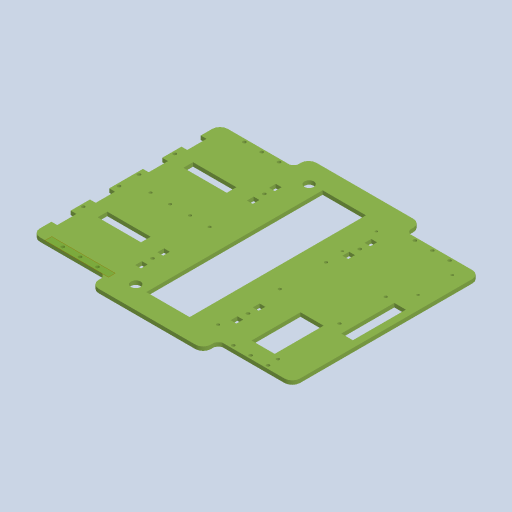
# Autodesk Inventor part: верхняя пластина
Saved by Autodesk Inventor 2024.2 (Build 282272000, 272)
## iProperties
Created: 2025-11-23
Part Number: верхняя пластина
Material: Типовые
Document SubType Name: Modeling
Designer: katya_notebook
Density: 1 g/cm^3
Appearance: Оливково-зеленый
Mass: 177.745 g
Surface Area: 959.322 cm^2
Volume: 177.745 cm^3
Author: katya_notebook
Autodesk Inventor part; units mm, degrees
ref_plane "YZ Plane" through (0, 0, 0) normal (1, 0, 0) x (0, 1, 0)
ref_plane "XZ Plane" through (0, 0, 0) normal (0, 1, 0) x (-1, 0, 0)
ref_plane "XY Plane" through (0, 0, 0) normal (0, 0, 1) x (1, 0, 0)
ref_plane "РабПлоскость1" through (-487.5503, -280.3956, -187.6025) normal (0, -1, 0) x (1, 0, 0)
sketch "Эскиз1" plane through (-487.5503, -280.3956, -187.6025) normal (0, -1, 0) x (1, 0, 0)
  line L0 (-76.4763, 6.5) -> (193.5237, 6.5)
  line L1 (193.5237, 6.5) -> (193.5237, -188.5)
  line L2 (193.5237, -188.5) -> (-76.4763, -188.5)
  line L3 (-76.4763, -188.5) -> (-76.4763, 6.5)
  line L4 (-76.4763, -13.5) -> (-76.4763, -1.5) projected
  circle A0 centre (-12, 3.25) radius 1.75
  circle A1 centre (-48, 3.25) radius 1.75
  circle A2 centre (-30, 3.25) radius 1.75
  line L5 (-76.4763, -91) -> (193.5237, -91)
  circle A3 centre (-12, -185.25) radius 1.75
  circle A4 centre (-48, -185.25) radius 1.75
  circle A5 centre (-30, -185.25) radius 1.75
  point P0 (487.5503, 187.6025)
  point P1 (-60, 3.25)
  dimension "d0" = 195
  dimension "d1" = 270
  dimension "d2" = 0
  dimension "d5" = 3.5
  dimension "d6" = 3.5
  dimension "d8" = 12
  dimension "d9" = 3.25
  dimension "d10" = 3.25
  dimension "d11" = 3.5
  dimension "d12" = 3.25
  dimension "d13" = 18
  dimension "d14" = 97.5
  constraints: 10 end point, 6 centre point, 3 symmetric about line, 2 parallel, 2 perpendicular, 1 horizontal, 1 midpoint, 1 point on line, 3 other
  measures "d0" distance of L0.end L1.end
  measures "d1" distance of L1.end L2.end
  measures "d2" distance between parallel lines of L4 L3
  measures "d5" diameter of A1
  measures "d6" diameter of A0
  measures "d8" distance of A1.centre point (-60, 3.25)
  measures "d9" distance from line of L0 A0.centre
  measures "d10" distance from line of L0 A1.centre
  measures "d11" diameter of A2
  measures "d12" distance from line of L0 A2.centre
  measures "d13" distance of A1.centre A2.centre
  measures "d14" distance between parallel lines of L5 L0
extrude "Выдавливание1" add sketch "Эскиз1" along normal blind 4 contours L0 L1 L5 L3 | L1 L2 L3 L5 | A0 | A1 | A2 | A3 | A4 | A5
sketch "Эскиз2" plane through (-487.5503, -284.3956, -187.6025) normal (0, -1, 0) x (1, 0, 0)
  circle A0 centre (-48, -185.25) radius 1.75 projected
  circle A1 centre (-30, -185.25) radius 1.75 projected
  circle A2 centre (-12, -185.25) radius 1.75 projected
  line L0 (0, -182) -> (-60, -182) projected
  line L1 (-60, -182) -> (-60, -188.5) projected
  line L2 (0, -188.5) -> (-60, -188.5) projected
  line L3 (0, -182) -> (0, -188.5) projected
  circle A3 centre (-48, 3.25) radius 1.75 projected
  circle A4 centre (-30, 3.25) radius 1.75 projected
  circle A5 centre (-12, 3.25) radius 1.75 projected
  line L4 (0, 0) -> (-60, 0) projected
  line L5 (0, 0) -> (0, 6.5) projected
  line L6 (0, 6.5) -> (-60, 6.5) projected
  line L7 (-60, 0) -> (-60, 6.5) projected
  circle A6 centre (165.0475, 3.25) radius 1.75 projected
  circle A7 centre (129.0475, 3.25) radius 1.75 projected
  circle A8 centre (147.0475, 3.25) radius 1.75 projected
  line L8 (116.803, 6.5) -> (116.803, 0) projected
  line L9 (116.803, 0) -> (176.803, 0) projected
  line L10 (176.803, 0) -> (176.803, 6.5) projected
  line L11 (176.803, 6.5) -> (116.803, 6.5) projected
  circle A9 centre (165.0475, -185.25) radius 1.75 projected
  circle A10 centre (129.0475, -185.25) radius 1.75 projected
  circle A11 centre (147.0475, -185.25) radius 1.75 projected
  line L12 (116.803, -188.5) -> (116.803, -182) projected
  line L13 (176.803, -188.5) -> (116.803, -188.5) projected
  line L14 (176.803, -182) -> (176.803, -188.5) projected
  line L15 (116.803, -182) -> (176.803, -182) projected
  line L16 (81.0237, 0.5) -> (81.0237, -182.5) projected
  line L17 (36.0237, 0.5) -> (81.0237, 0.5) projected
  line L18 (36.0237, -182.5) -> (36.0237, 0.5) projected
  line L19 (36.0237, -182.5) -> (81.0237, -182.5) projected
  point P0 (487.5503, 187.6025)
extrude "Выдавливание2" cut sketch "Эскиз2" against normal blind 10 contours A0 | A1 | A2 | A3 | A4 | A5 | A6 | A7 | A8 | A9 | A10 | A11
sketch "Эскиз3" plane through (-487.5503, -284.3956, -187.6025) normal (0, -1, 0) x (1, 0, 0)
  circle A0 centre (23.5237, -1) radius 5 projected
  circle A1 centre (23.5237, -181) radius 5 projected
  line L0 (36.0237, -182.5) -> (36.0237, 0.5) projected
  line L1 (81.0237, 0.5) -> (81.0237, -182.5) projected
  line L2 (36.0237, 0.5) -> (81.0237, 0.5) projected
  line L3 (81.0237, -182.5) -> (36.0237, -182.5) projected
  point P0 (487.5503, 187.6025)
extrude "Выдавливание3" cut sketch "Эскиз3" against normal blind 10
sketch "Эскиз4" plane through (-487.5503, -284.3956, -187.6025) normal (0, -1, 0) x (1, 0, 0)
  arc A0 (116.803, 10.7701) -> (120.803, 6.5) centre (124.2371, 13.7254) ccw projected
  line L0 (116.803, 10.7701) -> (0.2701, 10.7701) projected
  arc A1 (-4, 6.5) -> (0.2701, 10.7701) centre (-7.1034, 13.8735) ccw projected
  arc A2 (0, -192.5) -> (-4, -188.5) centre (-7.2915, -195.7915) ccw projected
  line L1 (0, -192.5) -> (116.803, -192.5) projected
  arc A3 (120.803, -188.5) -> (116.803, -192.5) centre (124.0945, -195.7915) ccw projected
  line L2 (120.803, -188.5) -> (-4, -188.5)
  line L3 (-4, 6.5) -> (120.803, 6.5)
  point P0 (487.5503, 187.6025)
  constraints: 4 end point, 1 horizontal, 1 parallel
extrude "Выдавливание4" add sketch "Эскиз4" against normal blind 4
sketch "Эскиз5" plane through (-487.5503, -284.3956, -187.6025) normal (0, -1, 0) x (1, 0, 0)
  line L0 (174.5237, -118.4235) -> (174.5237, -63.4235) projected
  line L1 (186.5237, -118.4235) -> (174.5237, -118.4235) projected
  line L2 (186.5237, -63.4235) -> (186.5237, -118.4235) projected
  line L3 (174.5237, -63.4235) -> (186.5237, -63.4235) projected
  point P0 (487.5503, 187.6025)
extrude "Выдавливание5" cut sketch "Эскиз5" against normal blind 10
ref_plane "РабПлоскость2" through (-558.0266, -285.3956, -376.1025) normal (1, 0, 0) x (0, 1, 0)
sketch "Эскиз7" plane through (-564.0266, -280.3956, -376.1025) normal (-1, 0, 0) x (0, 0, 1)
  line L0 (175, -5) -> (175, 0) projected
  line L1 (155, 0) -> (155, -5) projected
  line L2 (155, -5) -> (175, -5) projected
  line L3 (195, 0) -> (0, 0) projected
  line L4 (115, -5) -> (135, -5) projected
  line L5 (135, -5) -> (135, 0) projected
  line L6 (115, 0) -> (115, -5) projected
  line L7 (80, -5) -> (80, 0) projected
  line L8 (60, -5) -> (80, -5) projected
  line L9 (60, 0) -> (60, -5) projected
  line L10 (40, -5) -> (40, 0) projected
  line L11 (20, -5) -> (40, -5) projected
  line L12 (20, 0) -> (20, -5) projected
  line L13 (90.375, 55.705) -> (90.375, 55.205) projected
  line L14 (90.375, 55.205) -> (88.875, 55.205) projected
  line L15 (85.375, 55.205) -> (83.875, 55.205) projected
  line L16 (83.875, 55.205) -> (83.875, 55.705) projected
  line L17 (80, 59.705) -> (80, 60.705) projected
  line L18 (80, 60.705) -> (60, 60.705) projected
  line L19 (60, 60.705) -> (60, 59.705) projected
  line L20 (51.75, 55.205) -> (51.75, 47.705) projected
  line L21 (53.25, 55.705) -> (53.25, 55.205) projected
  line L22 (53.25, 55.205) -> (51.75, 55.205) projected
  line L23 (51.75, 47.705) -> (48.25, 47.705) projected
  line L24 (48.25, 47.705) -> (48.25, 55.205) projected
  line L25 (48.25, 55.205) -> (46.75, 55.205) projected
  line L26 (46.75, 55.205) -> (46.75, 55.705) projected
  line L27 (40, 59.705) -> (40, 60.705) projected
  line L28 (40, 60.705) -> (20, 60.705) projected
  line L29 (20, 60.705) -> (20, 59.705) projected
  line L30 (0, 59.705) -> (0, 0) projected
  line L31 (20, 0) -> (0, 0) projected
  line L32 (20, 0) -> (20, -5) projected
  line L33 (20, -5) -> (40, -5) projected
  line L34 (40, -5) -> (40, 0) projected
  line L35 (48.25, 0) -> (40, 0) projected
  line L36 (48.25, 0) -> (48.25, 1.5) projected
  line L37 (48.25, 1.5) -> (46.75, 1.5) projected
  line L38 (46.75, 1.5) -> (46.75, 4.5) projected
  line L39 (46.75, 4.5) -> (48.25, 4.5) projected
  line L40 (48.25, 4.5) -> (48.25, 12) projected
  line L41 (48.25, 12) -> (51.75, 12) projected
  line L42 (51.75, 12) -> (51.75, 4.5) projected
  line L43 (51.75, 4.5) -> (53.25, 4.5) projected
  line L44 (53.25, 4.5) -> (53.25, 1.5) projected
  line L45 (53.25, 1.5) -> (51.75, 1.5) projected
  line L46 (51.75, 1.5) -> (51.75, 0) projected
  line L47 (60, 0) -> (51.75, 0) projected
  line L48 (60, 0) -> (60, -5) projected
  line L49 (60, -5) -> (80, -5) projected
  line L50 (80, -5) -> (80, 0) projected
  line L51 (85.375, 0) -> (80, 0) projected
  line L52 (85.375, 0) -> (85.375, 1.5) projected
  line L53 (85.375, 1.5) -> (83.875, 1.5) projected
  line L54 (83.875, 1.5) -> (83.875, 4.5) projected
  line L55 (83.875, 4.5) -> (85.375, 4.5) projected
  line L56 (88.875, 1.5) -> (88.875, 0) projected
  line L57 (88.875, 4.5) -> (90.375, 4.5) projected
  line L58 (90.375, 4.5) -> (90.375, 1.5) projected
  line L59 (90.375, 1.5) -> (88.875, 1.5) projected
  line L60 (106.125, 0) -> (88.875, 0) projected
  line L61 (115, 0) -> (109.625, 0) projected
  line L62 (106.125, 0) -> (106.125, 1.5) projected
  line L63 (106.125, 1.5) -> (104.625, 1.5) projected
  line L64 (104.625, 1.5) -> (104.625, 4.5) projected
  line L65 (104.625, 4.5) -> (106.125, 4.5) projected
  line L66 (109.625, 1.5) -> (109.625, 0) projected
  line L67 (109.625, 4.5) -> (111.125, 4.5) projected
  line L68 (111.125, 4.5) -> (111.125, 1.5) projected
  line L69 (111.125, 1.5) -> (109.625, 1.5) projected
  line L70 (115, 0) -> (115, -5) projected
  line L71 (115, -5) -> (135, -5) projected
  line L72 (135, -5) -> (135, 0) projected
  line L73 (143.25, 0) -> (135, 0) projected
  line L74 (143.25, 0) -> (143.25, 1.5) projected
  line L75 (143.25, 1.5) -> (141.75, 1.5) projected
  line L76 (141.75, 1.5) -> (141.75, 4.5) projected
  line L77 (141.75, 4.5) -> (143.25, 4.5) projected
  line L78 (143.25, 4.5) -> (143.25, 12) projected
  line L79 (143.25, 12) -> (146.75, 12) projected
  line L80 (146.75, 12) -> (146.75, 4.5) projected
  line L81 (146.75, 4.5) -> (148.25, 4.5) projected
  line L82 (148.25, 4.5) -> (148.25, 1.5) projected
  line L83 (148.25, 1.5) -> (146.75, 1.5) projected
  line L84 (146.75, 1.5) -> (146.75, 0) projected
  line L85 (155, 0) -> (146.75, 0) projected
  line L86 (155, 0) -> (155, -5) projected
  line L87 (155, -5) -> (175, -5) projected
  line L88 (175, -5) -> (175, 0) projected
  line L89 (195, 0) -> (175, 0) projected
  line L90 (195, 59.705) -> (195, 0) projected
  line L91 (175, 59.705) -> (175, 60.705) projected
  line L92 (175, 60.705) -> (155, 60.705) projected
  line L93 (155, 60.705) -> (155, 59.705) projected
  line L94 (146.75, 55.205) -> (146.75, 47.705) projected
  line L95 (148.25, 55.705) -> (148.25, 55.205) projected
  line L96 (148.25, 55.205) -> (146.75, 55.205) projected
  line L97 (146.75, 47.705) -> (143.25, 47.705) projected
  line L98 (143.25, 47.705) -> (143.25, 55.205) projected
  line L99 (143.25, 55.205) -> (141.75, 55.205) projected
  line L100 (141.75, 55.205) -> (141.75, 55.705) projected
  line L101 (135, 59.705) -> (135, 60.705) projected
  line L102 (135, 60.705) -> (115, 60.705) projected
  line L103 (115, 60.705) -> (115, 59.705) projected
  line L104 (111.125, 55.705) -> (111.125, 55.205) projected
  line L105 (111.125, 55.205) -> (109.625, 55.205) projected
  line L106 (106.125, 55.205) -> (104.625, 55.205) projected
  line L107 (104.625, 55.205) -> (104.625, 55.705) projected
  line L108 (175, 55.705) -> (187, 55.705) projected
  line L109 (115, 55.705) -> (111.125, 55.705) projected
  line L110 (104.625, 55.705) -> (90.375, 55.705) projected
  line L111 (83.875, 55.705) -> (80, 55.705) projected
  line L112 (80, 55.705) -> (80, 59.705) projected
  line L113 (60, 59.705) -> (60, 55.705) projected
  line L114 (60, 55.705) -> (53.25, 55.705) projected
  line L115 (46.75, 55.705) -> (40, 55.705) projected
  line L116 (40, 55.705) -> (40, 59.705) projected
  line L117 (155, 59.705) -> (155, 55.705) projected
  line L118 (155, 55.705) -> (148.25, 55.705) projected
  line L119 (141.75, 55.705) -> (135, 55.705) projected
  line L120 (135, 55.705) -> (135, 59.705) projected
  line L121 (115, 59.705) -> (115, 55.705) projected
  line L122 (109.625, 55.205) -> (109.625, 47.705) projected
  line L123 (109.625, 47.705) -> (106.125, 47.705) projected
  line L124 (106.125, 47.705) -> (106.125, 55.205) projected
  line L125 (88.875, 55.205) -> (88.875, 47.705) projected
  line L126 (88.875, 47.705) -> (85.375, 47.705) projected
  line L127 (85.375, 47.705) -> (85.375, 53.705) projected
  line L128 (85.375, 6) -> (85.375, 12) projected
  line L129 (85.375, 12) -> (88.875, 12) projected
  line L130 (106.125, 4.5) -> (106.125, 12) projected
  line L131 (106.125, 12) -> (109.625, 12) projected
  line L132 (109.625, 12) -> (109.625, 4.5) projected
  line L133 (85.375, 6) -> (85.375, 6) projected
  line L134 (88.875, 12) -> (88.875, 4.5) projected
  line L135 (85.375, 53.705) -> (85.375, 53.705) projected
  line L136 (0, 59.705) -> (20, 59.705) projected
  line L137 (85.375, 4.5) -> (85.375, 6) projected
  line L138 (175, 59.705) -> (195, 59.705) projected
  line L139 (85.375, 53.705) -> (85.375, 55.205) projected
  point P0 (376.1025, 280.3956)
  point P1 (88.875, 49.205)
  point P2 (85.375, 49.205)
  point P3 (85.375, 9.5)
  point P4 (106.125, 9.5)
  point P5 (109.625, 9.5)
  point P6 (109.625, 6.5)
  point P7 (109.625, 49.205)
  point P8 (106.125, 49.205)
  point P9 (155, 55.705)
  point P10 (175, 55.705)
  point P11 (115, 55.705)
  point P12 (135, 55.705)
  point P13 (60, 55.705)
  point P14 (80, 55.705)
  point P15 (20, 55.705)
  point P16 (40, 55.705)
  point P17 (20, 0)
  point P18 (40, 0)
  point P19 (60, 0)
  point P20 (80, 0)
  point P21 (135, 0)
  point P22 (46.75, 47.1901)
  dimension "d0" = 195
  dimension "d1" = 270
  dimension "d2" = 0
  dimension "d5" = 3.5
  dimension "d6" = 3.5
  dimension "d8" = 12
  dimension "d9" = 3.25
  dimension "d10" = 3.25
  dimension "d11" = 3.5
  dimension "d12" = 3.25
  dimension "d13" = 18
  dimension "d14" = 97.5
extrude "Выдавливание7" cut sketch "Эскиз7" against normal up to surface (6 mm away) contours L2 L1 L3 L0 | L5 L4 L6 L3 | L7 L8 L9 L3 | L10 L11 L12 L3
sketch "Эскиз8" plane through (-487.5503, -284.3956, -187.6025) normal (0, -1, 0) x (1, 0, 0)
  line L0 (-70.4763, -45.25) -> (-76.4763, -45.25) projected
  line L1 (-76.4763, -40.25) -> (-70.4763, -40.25) projected
  line L2 (-76.4763, -45.25) -> (-76.4763, -41.75) projected
  line L3 (-76.4763, -45.25) -> (-70.4763, -45.25) projected
  line L4 (-70.4763, -41.75) -> (-70.4763, -45.25) projected
  line L5 (-76.4763, -41.75) -> (-70.4763, -41.75) projected
  line L6 (-76.4763, -103.125) -> (-76.4763, -103.125) projected
  line L7 (-76.4763, -103.125) -> (-70.4763, -103.125) projected
  line L8 (-70.4763, -103.125) -> (-70.4763, -103.125) projected
  line L9 (-76.4763, -140.25) -> (-76.4763, -136.75) projected
  line L10 (-76.4763, -140.25) -> (-70.4763, -140.25) projected
  line L11 (-70.4763, -136.75) -> (-70.4763, -140.25) projected
  line L12 (-76.4763, -136.75) -> (-70.4763, -136.75) projected
  circle A0 centre (-73.4763, -43.5) radius 1.75
  circle A1 centre (-73.4763, -80.625) radius 1.75
  circle A2 centre (-73.4763, -101.375) radius 1.75
  circle A3 centre (-73.4763, -138.5) radius 1.75
  line L13 (-76.4763, -103.125) -> (-70.4763, -103.125) projected
  point P0 (487.5503, 187.6025)
  constraints: 4 centre point
extrude "Выдавливание8" cut sketch "Эскиз8" against normal blind 10 contours A0 | A3 | A1 | A2
sketch "Эскиз9" plane through (-487.5503, -284.3956, -187.6025) normal (0, -1, 0) x (1, 0, 0)
  line L0 (0, -192.5) -> (116.803, -192.5) projected
  line L1 (0, -192.5) -> (0, -204)
  line L2 (0, -204) -> (116.803, -204)
  line L3 (116.803, -204) -> (116.803, -192.5)
  line L4 (0, -192.5) -> (116.803, -192.5)
  line L5 (116.803, 10.7701) -> (0.2701, 10.7701) projected
  line L6 (0.2701, 10.7701) -> (116.803, 10.7701)
  line L7 (116.803, 10.7701) -> (116.803, 22.2701)
  line L8 (116.803, 22.2701) -> (0.2701, 22.2701)
  line L9 (0.2701, 22.2701) -> (0.2701, 10.7701)
  point P0 (487.5503, 187.6025)
  point P1 (116.803, 10.7701)
  dimension "d29" = 11.5
  dimension "d30" = 11.5
  constraints: 16 end point, 3 perpendicular, 2 horizontal, 2 parallel, 1 vertical
  measures "d29" distance of L1.end L0.start
  measures "d30" distance of L6.end L7.end
extrude "Выдавливание9" add sketch "Эскиз9" against normal blind 4
fillet "Сопряжение1" radius 8 7 edges at (-487.2802, -282.3956, -165.3324) (-370.7474, -282.3956, -165.3324) (-294.0266, -282.3956, -181.1025) (-294.0266, -282.3956, -376.1025) (-370.7474, -282.3956, -391.6025) (-487.5503, -282.3956, -391.6025) (-564.0266, -282.3956, -376.1025)
fillet "Сопряжение2" radius 8 1 edges at (-564.0266, -282.3956, -181.1025)
sketch "Эскиз10" plane through (-487.5503, -284.3956, -187.6025) normal (0, -1, 0) x (1, 0, 0)
  line L0 (-56.4763, -130.5) -> (-11.4763, -130.5)
  line L1 (-11.4763, -130.5) -> (-11.4763, -140.5)
  line L2 (-11.4763, -140.5) -> (-56.4763, -140.5)
  line L3 (-56.4763, -140.5) -> (-56.4763, -130.5)
  line L4 (-56.4763, -41.5) -> (-11.4763, -41.5)
  line L5 (-11.4763, -41.5) -> (-11.4763, -51.5)
  line L6 (-11.4763, -51.5) -> (-56.4763, -51.5)
  line L7 (-56.4763, -51.5) -> (-56.4763, -41.5)
  line L8 (-68.4763, -188.5) -> (-4, -188.5) projected
  line L9 (-76.4763, -128.5) -> (-76.4763, -148.5) projected
  point P0 (487.5503, 187.6025)
  point P1 (-33.9763, -140.5)
  point P2 (-56.4763, -135.5)
  dimension "d35" = 10
  dimension "d36" = 48
  dimension "d37" = 89
  dimension "d38" = 10
  dimension "d39" = 45
  dimension "d40" = 20
  constraints: 16 end point, 4 parallel, 2 horizontal, 2 midpoint, 2 perpendicular, 2 point on line
  measures "d35" distance of L2.end L0.start
  measures "d36" distance from line of L8 point (-33.976, -140.5)
  measures "d37" distance between parallel lines of L0 L4
  measures "d38" distance of L6.end L4.start
  measures "d39" distance of L1.end L2.end
  measures "d40" distance from line of point (-56.476, -135.5) L9
extrude "Выдавливание10" cut sketch "Эскиз10" against normal blind 10
sketch "Эскиз11" plane through (-487.5503, -284.3956, -187.6025) normal (0, -1, 0) x (1, 0, 0)
  spline S0 degree 3 poles (8.7737, -90.9) (8.7737, -91.0887) (8.8115, -91.2898) (8.9647, -91.6592) (9.0801, -91.8277) (9.3461, -92.0936) (9.5145, -92.209) (9.884, -92.3622) (10.085, -92.4) (10.4625, -92.4) (10.6635, -92.3622) (11.033, -92.209) (11.2014, -92.0936) (11.4674, -91.8277) (11.5828, -91.6592) (11.7359, -91.2898) (11.7737, -91.0887) (11.7737, -90.7113) (11.7359, -90.5102) (11.5828, -90.1408) (11.4674, -89.9723) (11.2014, -89.7064) (11.033, -89.591) (10.6635, -89.4378) (10.4625, -89.4) (10.085, -89.4) (9.884, -89.4378) (9.5145, -89.591) (9.3461, -89.7064) (9.0801, -89.9723) (8.9647, -90.1408) (8.8115, -90.5102) (8.7737, -90.7113) (8.7737, -90.9) knots -0.905867 -0.905867 -0.905867 -0.905867 -0.84925 -0.84925 -0.792632 -0.792632 -0.736016 -0.736016 -0.6794 -0.6794 -0.622784 -0.622784 -0.566168 -0.566168 -0.509551 -0.509551 -0.452934 -0.452934 -0.396316 -0.396316 -0.339699 -0.339699 -0.283083 -0.283083 -0.226467 -0.226467 -0.169851 -0.169851 -0.113235 -0.113235 -0.056617 -0.056617 0 0 0 0 projected
  spline S1 degree 3 poles (-8.7263, -91.1) (-8.7263, -90.9113) (-8.7641, -90.7102) (-8.9172, -90.3408) (-9.0326, -90.1723) (-9.2986, -89.9064) (-9.467, -89.791) (-9.8365, -89.6378) (-10.0375, -89.6) (-10.415, -89.6) (-10.616, -89.6378) (-10.9855, -89.791) (-11.1539, -89.9064) (-11.4199, -90.1723) (-11.5353, -90.3408) (-11.6885, -90.7102) (-11.7263, -90.9113) (-11.7263, -91.2887) (-11.6885, -91.4898) (-11.5353, -91.8592) (-11.4199, -92.0277) (-11.1539, -92.2936) (-10.9855, -92.409) (-10.616, -92.5622) (-10.415, -92.6) (-10.0375, -92.6) (-9.8365, -92.5622) (-9.467, -92.409) (-9.2986, -92.2936) (-9.0326, -92.0277) (-8.9172, -91.8592) (-8.7641, -91.4898) (-8.7263, -91.2887) (-8.7263, -91.1) knots -0.905867 -0.905867 -0.905867 -0.905867 -0.84925 -0.84925 -0.792632 -0.792632 -0.736016 -0.736016 -0.6794 -0.6794 -0.622784 -0.622784 -0.566168 -0.566168 -0.509551 -0.509551 -0.452934 -0.452934 -0.396316 -0.396316 -0.339699 -0.339699 -0.283083 -0.283083 -0.226467 -0.226467 -0.169851 -0.169851 -0.113235 -0.113235 -0.056617 -0.056617 0 0 0 0 projected
  spline S2 degree 3 poles (-49.7263, -91.1) (-49.7263, -90.9113) (-49.7641, -90.7102) (-49.9172, -90.3408) (-50.0326, -90.1723) (-50.2986, -89.9064) (-50.467, -89.791) (-50.8365, -89.6378) (-51.0375, -89.6) (-51.415, -89.6) (-51.616, -89.6378) (-51.9855, -89.791) (-52.1539, -89.9064) (-52.4199, -90.1723) (-52.5353, -90.3408) (-52.6885, -90.7102) (-52.7263, -90.9113) (-52.7263, -91.2887) (-52.6885, -91.4898) (-52.5353, -91.8592) (-52.4199, -92.0277) (-52.1539, -92.2936) (-51.9855, -92.409) (-51.616, -92.5622) (-51.415, -92.6) (-51.0375, -92.6) (-50.8365, -92.5622) (-50.467, -92.409) (-50.2986, -92.2936) (-50.0326, -92.0277) (-49.9172, -91.8592) (-49.7641, -91.4898) (-49.7263, -91.2887) (-49.7263, -91.1) knots -0.905867 -0.905867 -0.905867 -0.905867 -0.84925 -0.84925 -0.792632 -0.792632 -0.736016 -0.736016 -0.6794 -0.6794 -0.622784 -0.622784 -0.566168 -0.566168 -0.509551 -0.509551 -0.452934 -0.452934 -0.396316 -0.396316 -0.339699 -0.339699 -0.283083 -0.283083 -0.226467 -0.226467 -0.169851 -0.169851 -0.113235 -0.113235 -0.056617 -0.056617 0 0 0 0 projected
  spline S3 degree 3 poles (-32.2263, -90.9) (-32.2263, -91.0887) (-32.1885, -91.2898) (-32.0353, -91.6592) (-31.9199, -91.8277) (-31.6539, -92.0936) (-31.4855, -92.209) (-31.116, -92.3622) (-30.915, -92.4) (-30.5375, -92.4) (-30.3365, -92.3622) (-29.967, -92.209) (-29.7986, -92.0936) (-29.5326, -91.8277) (-29.4172, -91.6592) (-29.2641, -91.2898) (-29.2263, -91.0887) (-29.2263, -90.7113) (-29.2641, -90.5102) (-29.4172, -90.1408) (-29.5326, -89.9723) (-29.7986, -89.7064) (-29.967, -89.591) (-30.3365, -89.4378) (-30.5375, -89.4) (-30.915, -89.4) (-31.116, -89.4378) (-31.4855, -89.591) (-31.6539, -89.7064) (-31.9199, -89.9723) (-32.0353, -90.1408) (-32.1885, -90.5102) (-32.2263, -90.7113) (-32.2263, -90.9) knots -0.905867 -0.905867 -0.905867 -0.905867 -0.84925 -0.84925 -0.792632 -0.792632 -0.736016 -0.736016 -0.6794 -0.6794 -0.622784 -0.622784 -0.566168 -0.566168 -0.509551 -0.509551 -0.452934 -0.452934 -0.396316 -0.396316 -0.339699 -0.339699 -0.283083 -0.283083 -0.226467 -0.226467 -0.169851 -0.169851 -0.113235 -0.113235 -0.056617 -0.056617 0 0 0 0 projected
  circle A0 centre (164.5237, -119.5) radius 1.6 projected
  circle A1 centre (164.5237, -71.5) radius 1.6 projected
  circle A2 centre (102.5237, -119.5) radius 1.6 projected
  circle A3 centre (102.5237, -71.5) radius 1.6 projected
  circle A4 centre (102.5237, -7.5) radius 1.6 projected
  circle A5 centre (164.5237, -7.5) radius 1.6 projected
  point P0 (487.5503, 187.6025)
  point P1 (8.7737, -90.9)
  point P2 (-8.7263, -91.1)
  point P3 (-49.7263, -91.1)
  point P4 (-32.2263, -90.9)
extrude "Выдавливание11" cut sketch "Эскиз11" against normal blind 10
sketch "Эскиз12" plane through (-487.5503, -284.3956, -187.6025) normal (0, -1, 0) x (1, 0, 0)
  circle A0 centre (179.4904, -173.5085) radius 1.3414 projected
  circle A1 centre (179.5461, -137.9824) radius 1.3005 projected
  circle A2 centre (100.9552, -137.9655) radius 1.2516 projected
  circle A3 centre (100.9111, -173.5023) radius 1.2859 projected
  point P0 (487.5503, 187.6025)
extrude "Выдавливание12" cut sketch "Эскиз12" against normal blind 10
sketch "Эскиз13" plane through (-487.5503, -284.3956, -187.6025) normal (0, -1, 0) x (1, 0, 0)
  line L0 (11.9631, -157) -> (11.9631, -164) projected
  line L1 (11.9631, -157) -> (5.9631, -157) projected
  line L2 (5.9631, -164) -> (5.9631, -157) projected
  line L3 (11.9631, -164) -> (5.9631, -164) projected
  line L4 (11.9631, -134) -> (11.9631, -141) projected
  line L5 (11.9631, -134) -> (5.9631, -134) projected
  line L6 (5.9631, -141) -> (5.9631, -134) projected
  line L7 (11.9631, -141) -> (5.9631, -141) projected
  line L8 (11.9631, -147.25) -> (11.9631, -150.75) projected
  line L9 (11.9631, -147.25) -> (5.9631, -147.25) projected
  line L10 (5.9631, -150.75) -> (5.9631, -147.25) projected
  line L11 (11.9631, -150.75) -> (5.9631, -150.75) projected
  circle A0 centre (8.9631, -149) radius 1.75
  line L12 (58.5237, -91) -> (-218.7393, -91)
  line L13 (58.5237, -91) -> (58.5237, -290.7211)
  line L14 (11.9631, -25) -> (11.9631, -18)
  line L15 (11.9631, -25) -> (5.9631, -25)
  line L16 (5.9631, -18) -> (5.9631, -25)
  line L17 (11.9631, -18) -> (5.9631, -18)
  line L18 (11.9631, -48) -> (11.9631, -41)
  line L19 (11.9631, -48) -> (5.9631, -48)
  line L20 (5.9631, -41) -> (5.9631, -48)
  line L21 (11.9631, -41) -> (5.9631, -41)
  line L22 (11.9631, -34.75) -> (11.9631, -31.25)
  line L23 (11.9631, -34.75) -> (5.9631, -34.75)
  line L24 (5.9631, -31.25) -> (5.9631, -34.75)
  line L25 (11.9631, -31.25) -> (5.9631, -31.25)
  circle A1 centre (8.9631, -33) radius 1.75
  line L26 (105.0844, -157) -> (105.0844, -164)
  line L27 (105.0844, -157) -> (111.0844, -157)
  line L28 (111.0844, -164) -> (111.0844, -157)
  line L29 (105.0844, -164) -> (111.0844, -164)
  line L30 (105.0844, -134) -> (105.0844, -141)
  line L31 (105.0844, -134) -> (111.0844, -134)
  line L32 (111.0844, -141) -> (111.0844, -134)
  line L33 (105.0844, -141) -> (111.0844, -141)
  line L34 (105.0844, -147.25) -> (105.0844, -150.75)
  line L35 (105.0844, -147.25) -> (111.0844, -147.25)
  line L36 (111.0844, -150.75) -> (111.0844, -147.25)
  line L37 (105.0844, -150.75) -> (111.0844, -150.75)
  circle A2 centre (108.0844, -149) radius 1.75
  line L38 (105.0844, -25) -> (105.0844, -18)
  line L39 (105.0844, -25) -> (111.0844, -25)
  line L40 (111.0844, -18) -> (111.0844, -25)
  line L41 (105.0844, -18) -> (111.0844, -18)
  line L42 (105.0844, -48) -> (105.0844, -41)
  line L43 (105.0844, -48) -> (111.0844, -48)
  line L44 (111.0844, -41) -> (111.0844, -48)
  line L45 (105.0844, -41) -> (111.0844, -41)
  line L46 (105.0844, -34.75) -> (105.0844, -31.25)
  line L47 (105.0844, -34.75) -> (111.0844, -34.75)
  line L48 (111.0844, -31.25) -> (111.0844, -34.75)
  line L49 (105.0844, -31.25) -> (111.0844, -31.25)
  circle A3 centre (108.0844, -33) radius 1.75
  point P0 (487.5503, 187.6025)
  constraints: 76 end point, 39 symmetric about line, 4 centre point, 1 horizontal, 1 vertical, 3 other
extrude "Выдавливание13" cut sketch "Эскиз13" against normal blind 10 contours L0 L3 L2 L1 | L4 L7 L6 L5 | A0 | L15 L16 L17 L14 | L19 L20 L21 L18 | A1 | L27 L28 L29 L26 | L31 L32 L33 L30 | A2 | L38 L41 L40 L39 | L42 L45 L44 L43 | A3
sketch "Эскиз14" plane through (-487.5503, -280.3956, -187.6025) normal (0, 1, 0) x (1, 0, 0)
  line L0 (136.2269, 59.341) -> (156.2269, 59.341) projected
  line L1 (156.2269, 12.591) -> (136.2269, 12.591) projected
  line L2 (134.2269, 61.341) -> (158.2269, 61.341)
  line L3 (158.2269, 61.341) -> (158.2269, 10.591)
  line L4 (158.2269, 10.591) -> (134.2269, 10.591)
  line L5 (134.2269, 10.591) -> (134.2269, 61.341)
  point P0 (487.5503, -187.6025)
  dimension "d49" = 2
  dimension "d50" = 2
  dimension "d51" = 2
  dimension "d52" = 2
  constraints: 8 end point, 2 parallel, 1 horizontal, 1 perpendicular
  measures "d49" horizontal distance of L2.start L0.start
  measures "d50" distance from line of L3 L0.end
  measures "d51" distance from line of L5 L0.start
  measures "d52" distance from line of L4 L1.end
extrude "Выдавливание14" cut sketch "Эскиз14" against normal blind 10
